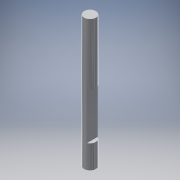
# Autodesk Inventor part: eje
Saved by Autodesk Inventor 2016 (Build 200138000, 138)
## iProperties
Created: 2016-09-08
Part Number: eje
Material: Aluminio 6061
Document SubType Name: Modeling
Designer: Iván
Density: 2.7 g/cm^3
Appearance: Aluminio - Plano
Author: Iván
Autodesk Inventor part; units mm, degrees
ref_plane "XZ Plane" through (0, 0, 0) normal (0, 1, 0) x (-1, 0, 0)
ref_plane "XY Plane" through (0, 0, 0) normal (0, 0, 1) x (1, 0, 0)
sketch "Boceto1" plane through (0, 0, 0) normal (0, 0, 1) x (1, 0, 0)
  circle A0 centre (0, 0) radius 2.5
  dimension "d0" = 5
  constraints: 1 centre point, 1 coincident
  measures "d0" diameter of A0
extrude "Extrusión1" add sketch "Boceto1" along normal blind 56
ref_plane "Plano de trabajo1" through (2.5, 0, 0) normal (1, 0, 0) x (0, 1, 0)
sketch "Boceto2" plane through (2.5, 0, 0) normal (1, 0, 0) x (0, 1, 0)
  line L0 (0, 0) -> (0, 10)
  line L1 (0, 10) -> (5.8177, 10)
  line L2 (5.8177, 10) -> (5.8177, 30)
  line L3 (0, 10) -> (-5.8625, 10)
  line L4 (-5.8625, 10) -> (-5.8625, 30)
  line L5 (-5.8625, 30) -> (5.8177, 30)
  dimension "d3" = 10
  dimension "d4" = 20
  constraints: 12 end point, 3 perpendicular, 2 vertical, 1 horizontal
  measures "d3" distance of L0.start L0.end
  measures "d4" distance of L1.end L2.end
extrude "Extrusión2" cut sketch "Boceto2" against normal blind 1.5
